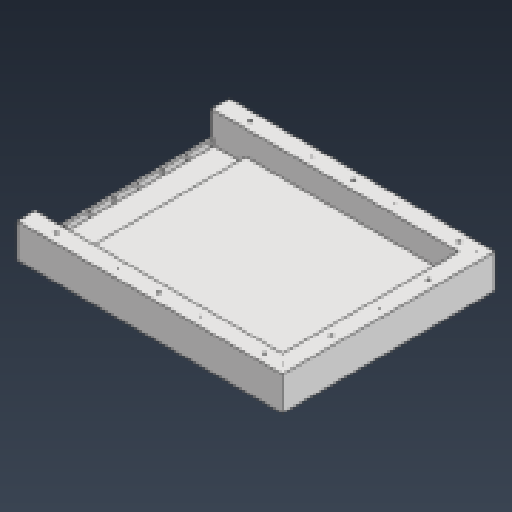
# Autodesk Inventor part: case0
Saved by Autodesk Inventor 2023 (Build 270158000, 158)
## iProperties
Created: 2026-01-23
Part Number: case0
Material: Generic
Document SubType Name: Modeling
Designer: szymo
Density: 1 g/cm^3
Appearance: Default
Author: szymo
Autodesk Inventor part; units mm, degrees
ref_plane "YZ Plane" through (0, 0, 0) normal (1, 0, 0) x (0, 1, 0)
ref_plane "XZ Plane" through (0, 0, 0) normal (0, 1, 0) x (-1, 0, 0)
ref_plane "XY Plane" through (0, 0, 0) normal (0, 0, 1) x (1, 0, 0)
sketch "Sketch1" plane through (0, 0, 0) normal (0, 1, 0) x (-1, 0, 0)
  line L0 (-37.4, -24.6) -> (-287.4, -24.6)
  line L1 (-287.4, -24.6) -> (-287.4, 175.4)
  line L2 (-287.4, 175.4) -> (-37.4, 175.4)
  line L3 (-37.4, 175.4) -> (-37.4, -24.6)
  line L4 (-37.4, -7.6) -> (-270.4, -7.6)
  line L5 (-270.4, -7.6) -> (-270.4, 158.4)
  line L6 (-270.4, 158.4) -> (-37.4, 158.4)
  line L7 (-244.2, 150.4) -> (-265.4, 150.4) projected
  line L8 (-265.4, 0.4) -> (-244.2, 0.4) projected
  line L9 (-265.4, 0.4) -> (-244.2, 0.4) projected
  point P0 (0, 0)
  dimension "d0" = 250
  dimension "d1" = 200
  dimension "offset_claw_nuts" = 17
  dimension "d3" = 17
  dimension "d4" = 17
  dimension "d5" = 8
  dimension "d6" = 8
  dimension "d7" = 5
  constraints: 14 end point, 3 perpendicular, 2 horizontal, 2 parallel, 2 point on line
  measures "d0" distance of L1.end L2.end
  measures "d1" distance of L0.end L1.end
  measures "offset_claw_nuts" distance between parallel lines of L0 L4
  measures "d3" distance between parallel lines of L1 L5
  measures "d4" distance between parallel lines of L2 L6
  measures "d5" distance between parallel lines of L4 L8
  measures "d6" distance between parallel lines of L6 L7
  measures "d7" distance from line of L5 L8.start
extrude "Extrusion1" add sketch "Sketch1" along normal blind 25 and the other way blind 7 contours L0 L1 L2 L3 L6 L5 L4
sketch "Sketch2" plane through (0, -7, 0) normal (0, -1, 0) x (1, 0, 0)
  line L0 (287.4, -24.6) -> (287.4, 175.4) projected
  line L1 (287.4, 175.4) -> (37.4, 175.4) projected
  line L2 (37.4, 175.4) -> (37.4, 158.4) projected
  line L3 (37.4, 158.4) -> (270.4, 158.4) projected
  line L4 (270.4, 158.4) -> (270.4, -7.6) projected
  line L5 (270.4, -7.6) -> (37.4, -7.6) projected
  line L6 (37.4, -7.6) -> (37.4, -24.6) projected
  line L7 (37.4, -24.6) -> (287.4, -24.6) projected
  line L8 (37.4, -24.6) -> (37.4, -24.6)
  line L9 (37.4, -24.6) -> (37.4, 175.4)
  line L10 (37.4, 175.4) -> (37.4, 175.4)
  line L11 (37.4, 175.4) -> (37.4, -24.6)
  point P0 (0, 0)
  point P1 (37.4, 158.4)
  point P2 (37.4, -7.6)
  constraints: 8 end point, 2 equal length, 1 horizontal, 1 perpendicular
extrude "Extrusion2" add sketch "Sketch2" against normal blind 3 contours L9 L3 L4 L5
sketch "Sketch3" plane through (37.4, -7, 175.4) normal (-1, 0, 0) x (0, 0, 1)
  line L0 (0, 0) -> (0, 32) projected
  line L1 (-17, 32) -> (0, 32) projected
  line L2 (-17, 3) -> (-17, 32) projected
  line L3 (-183, 3) -> (-17, 3) projected
  line L4 (-183, 3) -> (-183, 32) projected
  line L5 (-200, 32) -> (-183, 32) projected
  line L6 (-200, 0) -> (-200, 32) projected
  line L7 (0, 0) -> (-200, 0) projected
  line L8 (-183, 32) -> (-183, 32)
  line L9 (-183, 32) -> (-183, 32) construction
  line L10 (-183, 32) -> (-183, 9)
  line L11 (0, 32) -> (-200, 32) projected
  line L12 (-183, 9) -> (-17, 9)
  line L13 (-17, 9) -> (-17, 32)
  line L14 (-17, 32) -> (-17, 32)
  point P0 (-175.4, 7)
  point P1 (-75, 9)
  point P2 (-17, 9)
  dimension "d14" = 45
  dimension "d16" = 135
  dimension "d17" = 0
  dimension "d18" = 6
  dimension "d19" = 0
  dimension "d20" = 125
  dimension "d21" = 75
  constraints: 12 end point, 2 horizontal, 2 perpendicular, 1 equal length, 1 point on line
  measures "d14" angle of L8 L9
  measures "d16" angle of L13 L14
  measures "d17" distance between parallel lines of L4 L10
  measures "d18" distance between parallel lines of L3 L12
  measures "d19" distance between parallel lines of L13 L2
  measures "d20" distance from line of L6 point (-75, 9)
  measures "d21" distance from line of L0 point (-75, 9)
extrude "Extrusion3" add sketch "Sketch3" against normal blind 2.5 contours L2 L3 L4 L12
sketch "Sketch4" plane through (0, -4, 0) normal (0, 1, 0) x (1, 0, 0)
  line L0 (39.9, 7.6) -> (39.9, -158.4) projected
  line L1 (270.4, -158.4) -> (39.9, -158.4) projected
  line L2 (270.4, 7.6) -> (270.4, -158.4) projected
  line L3 (39.9, 7.6) -> (270.4, 7.6) projected
  line L4 (270.4, 7.6) -> (270.4, -158.4) projected
  line L5 (270.4, -158.4) -> (39.9, -158.4) projected
  line L6 (270.4, 7.6) -> (69.9, 7.6)
  line L7 (69.9, 7.6) -> (69.9, -158.4)
  line L8 (69.9, -158.4) -> (270.4, -158.4)
  line L9 (270.4, -158.4) -> (270.4, 7.6)
  point P0 (0, 0)
  point P1 (69.9, 7.6)
  point P2 (69.9, -158.4)
  dimension "d26" = 30
  constraints: 8 end point, 2 parallel, 1 horizontal, 1 perpendicular, 1 point on line
  measures "d26" distance between parallel lines of L7 L0
extrude "Extrusion4" add sketch "Sketch4" along normal up to surface (6 mm away) contours L3 L2 L1 L7
sketch "Sketch6" plane through (39.9, -7, 175.4) normal (1, 0, 0) x (0, 0, -1)
  line L0 (17, 3) -> (17, 9) projected
  line L1 (183, 3) -> (17, 3) projected
  line L2 (183, 9) -> (183, 3) projected
  line L3 (183, 9) -> (17, 9) projected
  circle A0 centre (20, 6) radius 3
  circle A1 centre (42.8571, 6) radius 3
  circle A2 centre (65.7143, 6) radius 3
  circle A3 centre (88.5714, 6) radius 3
  circle A4 centre (111.4286, 6) radius 3
  circle A5 centre (134.2857, 6) radius 3
  circle A6 centre (157.1429, 6) radius 3
  circle A7 centre (180, 6) radius 3
  point P0 (175.4, 7)
  dimension "d29" = 6
  dimension "d30" = 6
  dimension "d31" = 6
  dimension "d32" = 6
  dimension "d33" = 6
  dimension "d34" = 6
  dimension "d35" = 6
  dimension "d36" = 6
  dimension "d37" = 22.8571
  dimension "d38" = 22.8571
  dimension "d39" = 22.8571
  dimension "d40" = 22.8571
  dimension "d41" = 22.8571
  dimension "d42" = 22.8571
  dimension "d43" = 22.8571
  constraints: 10 tangent, 8 centre point
  measures "d29" diameter of A0
  measures "d30" diameter of A1
  measures "d31" diameter of A2
  measures "d32" diameter of A3
  measures "d33" diameter of A4
  measures "d34" diameter of A5
  measures "d35" diameter of A6
  measures "d36" diameter of A7
  measures "d37" distance of A1.centre A0.centre
  measures "d38" distance of A2.centre A1.centre
  measures "d39" distance of A3.centre A2.centre
  measures "d40" distance of A4.centre A3.centre
  measures "d41" distance of A5.centre A4.centre
  measures "d42" distance of A5.centre A6.centre
  measures "d43" distance of A6.centre A7.centre
hole "Hole1" at (39.9, -1, -4.6) at (39.9, -1, 18.2571) at (39.9, -1, 41.1143) at (39.9, -1, 63.9714) at (39.9, -1, 86.8286) at (39.9, -1, 132.5429) at (39.9, -1, 155.4) at (39.9, -1, 109.6857) direction (-1, 0, 0) diameter 3.6 end through all clearance for "Countersunk Flat Head Screw ISO 2009/7046" size "M3" standard "ISO"
sketch "Sketch7" plane through (0, 25, 0) normal (0, 1, 0) x (1, 0, 0)
  line L0 (287.4, -175.4) -> (287.4, 24.6) projected
  line L1 (287.4, 24.6) -> (37.4, 24.6) projected
  line L2 (37.4, 24.6) -> (37.4, 7.6) projected
  line L3 (37.4, 7.6) -> (270.4, 7.6) projected
  line L4 (270.4, 7.6) -> (270.4, -158.4) projected
  line L5 (270.4, -158.4) -> (37.4, -158.4) projected
  line L6 (37.4, -158.4) -> (37.4, -175.4) projected
  line L7 (37.4, -175.4) -> (287.4, -175.4) projected
  circle A0 centre (278.9, 16.1) radius 8.5
  circle A1 centre (278.9, -166.9) radius 8.5
  circle A2 centre (201.2333, 16.1) radius 8.5
  circle A3 centre (201.2333, -166.9) radius 8.5
  circle A4 centre (278.9, -75.4) radius 8.5
  circle A5 centre (123.5667, 16.1) radius 8.5
  circle A6 centre (123.5667, -166.9) radius 8.5
  circle A7 centre (45.9, 16.1) radius 8.5 construction
  circle A8 centre (45.9, -166.9) radius 8.5 construction
  point P0 (0, 0)
  dimension "d51" = 17
  dimension "d52" = 17
  dimension "d55" = 17
  dimension "d56" = 17
  dimension "d57" = 17
  dimension "d58" = 17
  dimension "d59" = 17
  dimension "d60" = 91.5
  dimension "d61" = 91.5
  dimension "d62" = 77.6667
  dimension "d63" = 77.6667
  dimension "d64" = 17
  dimension "d65" = 17
  dimension "d66" = 8.5
  dimension "d67" = 8.5
  dimension "d68" = 8.5
  dimension "d69" = 8.5
  dimension "d70" = 8.5
  dimension "d71" = 77.6667
  dimension "d72" = 77.6667
  dimension "d73" = 77.6667
  dimension "d74" = 77.6667
  dimension "d75" = 8.5
  constraints: 9 centre point, 7 tangent
  measures "d51" diameter of A1
  measures "d52" diameter of A0
  measures "d55" diameter of A2
  measures "d56" diameter of A3
  measures "d57" diameter of A4
  measures "d58" diameter of A5
  measures "d59" diameter of A6
  measures "d60" distance of A4.centre A0.centre
  measures "d61" distance of A1.centre A4.centre
  measures "d62" distance of A1.centre A3.centre
  measures "d63" distance of A6.centre A3.centre
  measures "d64" diameter of A7
  measures "d65" diameter of A8
  measures "d66" distance from line of L1 A5.centre
  measures "d67" distance from line of L1 A7.centre
  measures "d68" distance from line of L2 A7.centre
  measures "d69" distance from line of L6 A8.centre
  measures "d70" distance from line of L5 A8.centre
  measures "d71" distance of A8.centre A6.centre
  measures "d72" distance of A0.centre A2.centre
  measures "d73" distance of A5.centre A2.centre
  measures "d74" distance of A7.centre A5.centre
  measures "d75" distance from line of L5 A3.centre
hole "Hole2" at (123.5667, 25, -16.1) at (278.9, 25, -16.1) at (278.9, 25, 75.4) at (278.9, 25, 166.9) at (201.2333, 25, 166.9) at (201.2333, 25, -16.1) at (123.5667, 25, 166.9) direction (0, -1, 0) diameter 1 end through all
sketch "Sketch8" plane through (0, 25, 0) normal (0, 1, 0) x (1, 0, 0)
  circle A0 centre (201.2333, 16.1) radius 0.5 projected
  circle A1 centre (278.9, -166.9) radius 0.5 projected
  circle A2 centre (278.9, 16.1) radius 0.5 projected
  circle A3 centre (123.5667, 16.1) radius 0.5 projected
  circle A4 centre (278.9, -75.4) radius 0.5 projected
  circle A5 centre (201.2333, -166.9) radius 0.5 projected
  circle A6 centre (123.5667, -166.9) radius 0.5 projected
  line L0 (287.4, -175.4) -> (287.4, 24.6) projected
  line L1 (287.4, 24.6) -> (37.4, 24.6) projected
  line L2 (37.4, 24.6) -> (37.4, 7.6) projected
  line L3 (37.4, 7.6) -> (270.4, 7.6) projected
  line L4 (270.4, 7.6) -> (270.4, -158.4) projected
  line L5 (270.4, -158.4) -> (37.4, -158.4) projected
  line L6 (37.4, -158.4) -> (37.4, -175.4) projected
  line L7 (37.4, -175.4) -> (287.4, -175.4) projected
  circle A7 centre (65.9, 16.1) radius 8.5
  circle A8 centre (65.9, -166.9) radius 8.5
  circle A9 centre (278.9, -29.65) radius 8.5
  circle A10 centre (278.9, -121.15) radius 8.5
  circle A11 centre (261.9, 16.1) radius 8.5
  circle A12 centre (261.9, -166.9) radius 8.5
  circle A13 centre (162.4, 16.1) radius 8.5
  circle A14 centre (162.4, -166.9) radius 8.5
  line L8 (37.4, 24.6) -> (287.4, 24.6) projected
  line L9 (270.4, 7.6) -> (270.4, -158.4) projected
  line L10 (270.4, 24.6) -> (270.4, 7.6)
  line L11 (270.4, -158.4) -> (270.4, -175.4)
  point P0 (0, 0)
  dimension "d83" = 17
  dimension "d84" = 17
  dimension "d85" = 45.75
  dimension "d86" = 45.75
  dimension "d87" = 45.75
  dimension "d88" = 38.8333
  dimension "d89" = 38.8333
  dimension "d90" = 38.8333
  dimension "d91" = 38.8333
  dimension "d92" = 28.5
  dimension "d93" = 0
  constraints: 16 tangent, 8 centre point, 4 end point, 2 point on line, 1 collinear, 1 perpendicular
  measures "d83" diameter of A7
  measures "d84" diameter of A8
  measures "d85" distance of A9.centre A4.centre
  measures "d86" distance of A10.centre A4.centre
  measures "d87" distance of A2.centre A9.centre
  measures "d88" distance of A0.centre A13.centre
  measures "d89" distance of A3.centre A13.centre
  measures "d90" distance of A5.centre A14.centre
  measures "d91" distance of A6.centre A14.centre
  measures "d92" distance from line of L2 A7.centre
  measures "d93" horizontal distance of A8.centre A7.centre
hole "Hole3" at (261.9, 25, -16.1) at (278.9, 25, 29.65) at (278.9, 25, 121.15) at (261.9, 25, 166.9) at (162.4, 25, -16.1) at (65.9, 25, -16.1) at (65.9, 25, 166.9) at (162.4, 25, 166.9) direction (0, -1, 0) diameter 3 end through all
equation "\"d3\" = offset_claw_nuts"
equation "\"d4\" = offset_claw_nuts"
equation "\"d6\" = d5"
equation "\"d37\" = d43"
equation "\"d38\" = d43"
equation "\"d39\" = d43"
equation "\"d40\" = d43"
equation "\"d41\" = d43"
equation "\"d42\" = d43"
equation "\"d60\" = d61"
equation "\"d62\" = d71"
equation "\"d63\" = d71"
equation "\"d66\" = 0.5 * d58"
equation "\"d67\" = 0.5 * d64"
equation "\"d68\" = 0.5 * d64"
equation "\"d69\" = 0.5 * d65"
equation "\"d70\" = 0.5 * d65"
equation "\"d72\" = d74"
equation "\"d73\" = d74"
body "Solid1"
